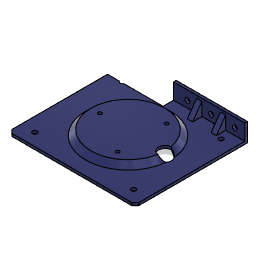
Case_bottom v23 (Autodesk Fusion 360 design; units mm, degrees)
Autodesk Fusion 360 part; units mm, degrees
sketch "Sketch1" plane through (0, 0, 0) normal (0, 0, 1) x (1, 0, 0)
  line L0 (0, 0) -> (54, 0)
  line L1 (54, 0) -> (54, 14)
  line L2 (54, 14) -> (0, 14)
  line L3 (0, 14) -> (0, 0)
  line L4 (0, 7) -> (54, 7) construction
  circle A0 centre (46.5, 7) radius 1.9
  circle A1 centre (28.5, 7) radius 1.9
  circle A2 centre (10.5, 7) radius 1.9
  dimension "d1" = 54
  dimension "d2" = 14
  dimension "d3" = 3.8
  dimension "d4" = 3.8
  dimension "d5" = 3.8
  dimension "d6" = 7.5
  dimension "d7" = 18
  dimension "d8" = 18
  constraint horizontal L0
  constraint vertical L1
  constraint horizontal L2
  constraint vertical L3
  constraint coincident L0.start L3.end
  constraint midpoint L3 L4.start
  constraint midpoint L1 L4.end
  constraint coincident L4 A0.centre
  constraint coincident L4 A1.centre
  constraint coincident L4 A2.centre
  measures "d1" distance of L0.start L0.end
  measures "d2" distance of L0.start L2.end
  measures "d3" diameter of A0
  measures "d4" diameter of A1
  measures "d5" diameter of A2
  measures "d6" distance of L1 A0.centre
  measures "d7" distance of A0.centre A1.centre
  measures "d8" distance of A1.centre A2.centre
extrude "Extrude1" add sketch "Sketch1" along normal blind 2
sketch "Sketch2" plane through (0, 0, 0) normal (0, -1, 0) x (1, 0, 0)
  line L0 (0, 0) -> (54, 0)
  line L1 (54, 0) -> (54, 2)
  line L2 (54, 2) -> (0, 2)
  line L3 (0, 2) -> (0, 0)
  line L4 (54, 0) -> (-42, 0)
  line L5 (-42, 0) -> (-42, 85)
  line L6 (-42, 85) -> (54, 85)
  line L7 (54, 85) -> (54, 0)
  dimension "d11" = 96
  dimension "d14" = 85
  constraint horizontal L4
  constraint vertical L5
  constraint horizontal L6
  constraint vertical L7
  constraint coincident L0.end L1.start
  measures "d11" distance of L5.end L6.end
  measures "d14" distance of L4.end L5.end
extrude "Extrude2" add sketch "Sketch2" against normal blind 2
sketch "Sketch3" plane through (0, 2, 0) normal (0, 1, 0) x (-1, 0, 0)
  line L0 (-54, 2) -> (0, 2)
  line L1 (0, 2) -> (0, 0)
  line L2 (0, 0) -> (42, 0)
  line L3 (42, 0) -> (42, 85)
  line L4 (42, 85) -> (-54, 85)
  line L5 (-54, 85) -> (-54, 2)
  line L6 (-54, 85) -> (42, 0) construction
  line L7 (42, 85) -> (-54, 0) construction
  circle A0 centre (-6, 42.5) radius 21.362 construction
  circle A1 centre (-16.681, 24) radius 1.35
  circle A2 centre (-16.681, 61) radius 1.35
  circle A3 centre (15.362, 42.5) radius 1.35
  line L8 (-16.681, 24) -> (-16.681, 61) construction
  line L9 (15.362, 42.5) -> (-6, 42.5) construction
  line L10 (15.362, 42.5) -> (-16.681, 24) construction
  circle A4 centre (-34, 42.5) radius 5
  circle A5 centre (31.4349, 75.6455) radius 1.75
  line L11 (-6, 42.5) -> (-6, 21.138) construction
  circle A6 centre (31.4349, 9.3545) radius 1.75
  circle A7 centre (-43.4349, 9.3545) radius 1.75
  circle A8 centre (-43.4349, 75.6455) radius 1.75
  line L12 (-6, 42.5) -> (-34, 42.5) construction
  circle A9 centre (-6, 42.5) radius 28
  point P0 (-54, 0)
  point P1 (-6, 42.5)
  dimension "d15" = 2.7
  dimension "d16" = 2.7
  dimension "d17" = 2.7
  dimension "d18" = 37
  dimension "d20" = 37
  dimension "d22" = 28
  dimension "d23" = 10
  dimension "d26" = 3.5
  dimension "d27" = 50
  constraint coincident L4.end L5.start
  constraint coincident L2.end L3.start
  constraint coincident L3.end L4.start
  constraint coincident P0 L7.end
  constraint midpoint L6 P1
  constraint coincident P1 A0.centre
  constraint coincident A0 A1.centre
  constraint coincident A0 A2.centre
  constraint coincident A0 A3.centre
  constraint coincident A1.centre L8.start
  constraint coincident A2.centre L8.end
  constraint vertical L8
  constraint coincident A3.centre L9.start
  constraint horizontal L9
  constraint coincident L7 A5.centre
  constraint coincident A0 L11.end
  constraint perpendicular L9 L11
  constraint symmetric L9 A5 A6
  constraint symmetric A5 L11 A8
  constraint symmetric L11 A6 A7
  constraint coincident A4.centre L12.end
  constraint horizontal L12
  constraint coincident A4.centre A9
  measures "d15" diameter of A1
  measures "d16" diameter of A2
  measures "d17" diameter of A3
  measures "d18" distance of A1.centre A2.centre
  measures "d20" distance of A3.centre A1.centre
  measures "d22" distance of P1 A4.centre
  measures "d23" diameter of A4
  measures "d26" diameter of A5
  measures "d27" distance of P1 A5.centre
extrude "Extrude4" add sketch "Sketch3" along normal blind 4 contours A4 A9 picked at (-6, 42.5)
extrude "Extrude3" cut sketch "Sketch3" against normal through all contours A1 | A2 | A3 | A4 A9 | A4 A9 | A5 | A6 | A7 | A8 picked at (-32.3002, 42.5) picked at (-35.6292, 42.3798)
chamfer "Chamfer3" distance 2.5 angle 45 2 edges at (-42, 1, 85) (54, 1, 85)
chamfer "Chamfer1" distance 4 angle 45 1 edges at (-22, 2, 42.5)
sketch "Sketch4" plane through (0, 0, 0) normal (0, -1, 0) x (1, 0, 0)
  line L0 (51.5, 85) -> (-39.5, 85)
  line L1 (-42, 82.5) -> (-42, 0)
  line L2 (-42, 0) -> (54, 0)
  line L3 (54, 0) -> (54, 82.5)
  circle A0 centre (-31.4349, 9.3545) radius 1.75
  circle A1 centre (16.681, 61) radius 1.35
  circle A2 centre (-15.362, 42.5) radius 1.35
  circle A3 centre (43.4349, 9.3545) radius 1.75
  circle A4 centre (-31.4349, 75.6455) radius 1.75
  circle A5 centre (34, 42.5) radius 5
  circle A6 centre (16.681, 24) radius 1.35
  circle A7 centre (43.4349, 75.6455) radius 1.75
  line L4 (6, 0) -> (6, 85) construction
  line L5 (6, 42.5) -> (54, 42.5) construction
  circle A8 centre (6, 42.5) radius 28
  line L6 (54, 82.5) -> (51.5, 85)
  line L7 (-39.5, 85) -> (-42, 82.5)
  dimension "d31" = 56
  constraint midpoint L2 L4.start
  constraint midpoint L0 L4.end
  constraint midpoint L4 L5.start
  constraint coincident L3 L5.end
  constraint perpendicular L3 L5
  constraint coincident L5.start A8.centre
  measures "d31" diameter of A8
extrude "Extrude5" cut sketch "Sketch4" against normal blind 4 contours A5 A8 picked at (6, 42.5)
chamfer "Chamfer2" distance 4 angle 45 1 edges at (-22, 0, 42.5)
sketch "Sketch5" plane through (0, 0, 2) normal (0, 0, 1) x (1, 0, 0)
  line L0 (0, 2) -> (54, 2)
  line L1 (54, 2) -> (54, 14)
  line L2 (54, 14) -> (0, 14)
  line L3 (0, 14) -> (0, 2)
  circle A0 centre (46.5, 7) radius 1.9
  circle A1 centre (28.5, 7) radius 1.9
  circle A2 centre (10.5, 7) radius 1.9
  line L4 (10.5, 7) -> (28.5, 7) construction
  line L5 (28.5, 7) -> (46.5, 7) construction
  line L6 (21.5, 2) -> (17.5, 2)
  line L7 (17.5, 2) -> (17.5, 12)
  line L8 (17.5, 12) -> (21.5, 12)
  line L9 (21.5, 12) -> (21.5, 2)
  line L10 (21.5, 2) -> (17.5, 12) construction
  line L11 (17.5, 2) -> (21.5, 12) construction
  line L12 (39.5, 2) -> (35.5, 2)
  line L13 (35.5, 2) -> (35.5, 12)
  line L14 (35.5, 12) -> (39.5, 12)
  line L15 (39.5, 12) -> (39.5, 2)
  line L16 (39.5, 2) -> (35.5, 12) construction
  line L17 (35.5, 2) -> (39.5, 12) construction
  point P0 (19.5, 7)
  point P1 (37.5, 7)
  dimension "d36" = 4
  dimension "d37" = 4
  constraint coincident A2.centre L4.start
  constraint coincident A1.centre L4.end
  constraint coincident A0.centre L5.end
  constraint horizontal L6
  constraint perpendicular L6 L7
  constraint parallel L6 L8
  constraint parallel L7 L9
  constraint coincident L10 P0
  constraint coincident L11 P0
  constraint midpoint L4 P0
  constraint horizontal L12
  constraint perpendicular L12 L13
  constraint parallel L12 L14
  constraint parallel L13 L15
  constraint coincident L0 L12.start
  constraint coincident L16 P1
  constraint coincident L17 P1
  constraint midpoint L5 P1
  constraint collinear L6 L12
  measures "d36" distance of L7.end L8.end
  measures "d37" distance of L13.end L14.end
extrude "Extrude6" add sketch "Sketch5" along normal blind 7 contours L0 L6 L7 L8 L9 | L0 L12 L13 L14 L15
chamfer "Chamfer4" distance 10 distance2 7 2 edges at (19.5, 12, 9) (37.5, 12, 9) measured on face at (20.1667, 5.3333, 9) measured on face at (36.8333, 5.3333, 9)
sketch "Sketch7" plane through (0, 2, 0) normal (0, 1, 0) x (-1, 0, 0)
  line L0 (-35.5, 9) -> (-35.5, 2)
  line L1 (-35.5, 2) -> (-21.5, 2)
  line L2 (0, 2) -> (0, 0)
  line L3 (0, 0) -> (42, 0)
  line L4 (42, 0) -> (42, 82.5)
  line L5 (42, 82.5) -> (39.5, 85)
  line L6 (39.5, 85) -> (-51.5, 85)
  line L7 (-51.5, 85) -> (-54, 82.5)
  line L8 (-54, 82.5) -> (-54, 2)
  line L9 (-54, 2) -> (-39.5, 2)
  line L10 (-39.5, 2) -> (-39.5, 9)
  arc A0 (-37.8393, 39.2969) -> (-37.8393, 45.7031) centre (-6, 42.5) ccw
  arc A1 (-37.8393, 45.7031) -> (-37.8393, 39.2969) centre (-34, 42.5) ccw
  circle A2 centre (-43.4349, 75.6455) radius 1.75
  circle A3 centre (31.4349, 75.6455) radius 1.75
  circle A4 centre (-43.4349, 9.3545) radius 1.75
  circle A5 centre (31.4349, 9.3545) radius 1.75
  line L11 (42, 0) -> (0, 0)
  line L12 (0, 0) -> (0, 10)
  line L13 (0, 10) -> (42, 10)
  line L14 (42, 10) -> (42, 0)
  line L15 (-21.5, 2) -> (-21.5, 9)
  line L16 (-17.5, 9) -> (-17.5, 2)
  line L17 (-21.5, 9) -> (-17.5, 9)
  line L18 (-17.5, 2) -> (0, 2)
  line L19 (-39.5, 9) -> (-35.5, 9)
  dimension "d49" = 10
  constraint horizontal L11
  constraint vertical L12
  constraint horizontal L13
  constraint vertical L14
  constraint coincident L3.end L4.start
  constraint collinear L2 L12
  measures "d49" distance of L3.end L13.end
extrude "Extrude7" cut sketch "Sketch7" against normal through all contours L2 L3 L4 A5 L11 L12 L13 L14
